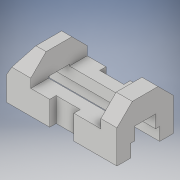
# Autodesk Inventor part: 410571040-2
Saved by Autodesk Inventor 2017 (Build 210142000, 142)
## iProperties
Part Number: 410571040-2
Material: 一般
Document SubType Name: Modeling
Designer: user
Density: 1 g/cm^3
Appearance: 預設
Author: user
Autodesk Inventor part; units mm, degrees
ref_plane "YZ Plane" through (0, 0, 0) normal (1, 0, 0) x (0, 1, 0)
ref_plane "XZ Plane" through (0, 0, 0) normal (0, 1, 0) x (-1, 0, 0)
ref_plane "XY Plane" through (0, 0, 0) normal (0, 0, 1) x (1, 0, 0)
sketch "草圖1" plane through (0, 0, 0) normal (1, 0, 0) x (0, 1, 0)
  line L0 (-32, 35) -> (9, 35)
  line L1 (9, 35) -> (28, 16)
  line L2 (28, 16) -> (28, 0)
  line L3 (-32, 35) -> (-32, 18)
  line L4 (-32, 18) -> (-16, 18)
  line L5 (-16, 18) -> (-16, 13)
  line L6 (-16, 13) -> (0, 13)
  line L7 (0, 13) -> (0, 6.0328)
  line L8 (28, 0) -> (52.708, 0)
  line L9 (-32, -35) -> (9, -35)
  line L10 (9, -35) -> (28, -16)
  line L11 (28, -16) -> (28, 0)
  line L12 (-32, -35) -> (-32, -18)
  line L13 (-32, -18) -> (-16, -18)
  line L14 (-16, -18) -> (-16, -13)
  line L15 (-16, -13) -> (0, -13)
  line L16 (0, -13) -> (0, 6.0328)
  point P0 (0, 0)
  dimension "d0" = 19
  dimension "d1" = 70
  dimension "d2" = 26
  dimension "d3" = 36
  dimension "d4" = 32
  dimension "d5" = 60
  dimension "d6" = 16
  dimension "d7" = 0
  dimension "d8" = 19
  constraints: 34 end point, 7 symmetric about line, 5 perpendicular, 2 horizontal, 1 point on line, 1 vertical
  measures "d0" horizontal distance of L1.end L0.end
  measures "d1" distance between parallel lines of L9 L0
  measures "d2" distance of L6.end L15.end
  measures "d3" distance between parallel lines of L13 L4
  measures "d4" distance from line of L12 L15.end
  measures "d5" distance between parallel lines of L3 L2
  measures "d6" distance of L3.end L4.end
  measures "d7" distance from line of point (0, 0) L16
  measures "d8" horizontal distance of L1.end L0.end
extrude "擠出1" add sketch "草圖1" against normal blind 137
sketch "草圖2" plane through (0, -32, 35) normal (0, 0, 1) x (1, 0, 0)
  line L0 (-137, 0) -> (-137, 41) projected
  line L1 (-137, 30) -> (-119.6795, 60)
  line L2 (0, 60) -> (-137, 60) projected
  line L3 (-137, 60) -> (-137, 30)
  line L4 (-119.6795, 60) -> (-137, 60)
  point P0 (0, 32)
  dimension "d12" = 30
  dimension "d13" = 30
  constraints: 6 end point, 2 point on line, 1 collinear, 1 vertical
  measures "d12" distance of L2.end L1.start
  measures "d13" angle of L3 L1
extrude "擠出2" cut sketch "草圖2" against normal blind 137
sketch "草圖3" plane through (0, -32, 35) normal (0, 0, 1) x (1, 0, 0)
  line L0 (0, 60) -> (-119.6795, 60) projected
  line L1 (-107, 60) -> (-20, 60)
  line L2 (-20, 60) -> (-20, 30)
  line L3 (-20, 30) -> (-107, 30)
  line L4 (-107, 30) -> (-107, 60)
  line L5 (-137, 0) -> (-137, 30) projected
  point P0 (0, 32)
  dimension "d16" = 30
  dimension "d17" = 30
  dimension "d18" = 87
  constraints: 8 end point, 2 parallel, 1 horizontal, 1 perpendicular, 1 point on line
  measures "d16" distance between parallel lines of L4 L5
  measures "d17" distance between parallel lines of L0 L3
  measures "d18" distance of L2.end L3.end
extrude "擠出3" cut sketch "草圖3" against normal blind 137
sketch "草圖4" plane through (-107, -2, 35) normal (0, 1, 0) x (1, 0, 0)
  line L0 (87, 0) -> (0, 0) projected
  line L1 (23.5, 0) -> (53.5, 0)
  line L2 (53.5, 0) -> (53.5, 8)
  line L3 (53.5, 8) -> (23.5, 8)
  line L4 (23.5, 8) -> (23.5, 0)
  line L5 (107, 70) -> (-30, 70) projected
  line L6 (23.5, 70) -> (53.5, 70)
  line L7 (53.5, 70) -> (53.5, 62)
  line L8 (53.5, 62) -> (23.5, 62)
  line L9 (23.5, 62) -> (23.5, 70)
  line L10 (-30, 0) -> (-30, 22) projected
  line L11 (-30, 48) -> (-30, 70) projected
  point P0 (107, 35)
  dimension "d21" = 53.5
  dimension "d22" = 53.5
  dimension "d23" = 30
  dimension "d24" = 30
  dimension "d25" = 8
  dimension "d26" = 8
  constraints: 16 end point, 4 parallel, 2 horizontal, 2 perpendicular, 2 point on line
  measures "d21" distance between parallel lines of L4 L10
  measures "d22" distance between parallel lines of L11 L9
  measures "d23" distance of L7.end L8.end
  measures "d24" distance of L2.end L3.end
  measures "d25" distance of L1.end L2.end
  measures "d26" distance of L6.end L7.end
extrude "擠出4" cut sketch "草圖4" against normal blind 137
